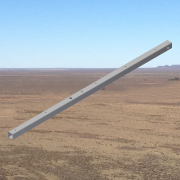
# Autodesk Inventor part: 2f2al
Saved by Autodesk Inventor 2014 SP1 (Build 180222100, 222)
## iProperties
Company: HERA Project
Created: 2013-06-27
Part Number: 2f2al
Material: Steel
Description: Feed backplane support crosspiece
Document SubType Name: Modeling
Designer: David DeBoer
Mass: 345.097 g
Surface Area: 540.887 cm^2
Volume: 43.9614 cm^3
Density: 7.85 g/cm^3
Appearance: Steel
Title: Feed backplane cross
Author: David DeBoer
Autodesk Inventor part; units mm, degrees
ref_plane "YZ Plane" through (0, 0, 0) normal (1, 0, 0) x (0, 1, 0)
ref_plane "XZ Plane" through (0, 0, 0) normal (0, 1, 0) x (-1, 0, 0)
ref_plane "XY Plane" through (0, 0, 0) normal (0, 0, 1) x (1, 0, 0)
sketch "Sketch1" plane through (0, 0, 0) normal (0, 0, 1) x (1, 0, 0)
  line L0 (3.175, 0) -> (22.225, 0)
  line L1 (25.4, 3.175) -> (25.4, 22.225)
  line L2 (22.225, 25.4) -> (3.175, 25.4)
  line L3 (0, 22.225) -> (0, 3.175)
  arc A0 (3.175, 25.4) -> (0, 22.225) centre (3.175, 22.225) ccw
  arc A1 (0, 3.175) -> (3.175, 0) centre (3.175, 3.175) ccw
  arc A2 (22.225, 0) -> (25.4, 3.175) centre (22.225, 3.175) ccw
  arc A3 (25.4, 22.225) -> (22.225, 25.4) centre (22.225, 22.225) ccw
  line L4 (3.175, 23.4) -> (22.225, 23.4)
  arc A4 (23.4, 22.225) -> (22.225, 23.4) centre (22.225, 22.225) ccw
  line L5 (23.4, 22.225) -> (23.4, 3.175)
  arc A5 (22.225, 2) -> (23.4, 3.175) centre (22.225, 3.175) ccw
  line L6 (22.225, 2) -> (3.175, 2)
  arc A6 (2, 3.175) -> (3.175, 2) centre (3.175, 3.175) ccw
  line L7 (2, 3.175) -> (2, 22.225)
  arc A7 (3.175, 23.4) -> (2, 22.225) centre (3.175, 22.225) ccw
  point P0 (0, 0)
  point P1 (25.4, 0)
  point P2 (0, 25.4)
  dimension "d0" = 25.4
  dimension "d1" = 25.4
  dimension "d2" = 3.175
  dimension "d3" = 2
  constraints: 16 end point, 16 point on circle, 8 centre point, 8 tangent, 6 point on line, 4 parallel, 3 equal radius, 2 perpendicular, 1 horizontal, 7 other
  measures "d0" distance of point (0, 0) point (25.4, 0)
  measures "d1" distance of point (0, 25.4) point (0, 0)
  measures "d2" radius of A0
  measures "d3" distance between parallel lines of L4 L2
extrude "Extrusion1" add sketch "Sketch1" along normal blind 1000
sketch "Sketch11" plane through (3.175, 25.4, 1000) normal (0, 1, 0) x (1, 0, 0)
  circle A0 centre (9.525, 500) radius 4.7917
  point P0 (-3.175, 1000)
  constraints: 1 centre point
hole "centerHole" at (12.7, 25.4, 500) direction (0, -1, 0) diameter 11 end through all clearance for "Flat Head Machine Screw" size "M10" standard "Ansi Metric M Profile"
sketch "Sketch12" plane through (3.175, 25.4, 1000) normal (0, 1, 0) x (1, 0, 0)
  line L0 (0, 1000) -> (0, 0) projected
  circle A0 centre (9.525, 927) radius 1.5875
  circle A1 centre (9.525, 777) radius 1.5875
  circle A2 centre (9.525, 627) radius 1.5875
  circle A3 centre (9.525, 500) radius 5.5 projected
  point P0 (-3.175, 1000)
  dimension "d76" = 3.175
  dimension "d80" = 150
  dimension "d140" = 127
  constraints: 3 centre point, 1 vertical, 4 other
  measures "d76" diameter of A0
  measures "d80" distance of A0.centre A1.centre
  measures "d140" distance of A2.centre A3.centre
hole "longSideHoles" at (12.7, 25.4, 73) at (12.7, 25.4, 223) at (12.7, 25.4, 373) direction (0, -1, 0) diameter 4.5 end through all clearance for "Flat Head Machine Screw" size "M4" standard "Ansi Metric M Profile"
sketch "Sketch13" plane through (3.175, 25.4, 1000) normal (0, 1, 0) x (1, 0, 0)
  line L0 (0, 1000) -> (0, 0) projected
  circle A0 centre (9.525, 68.2) radius 1.5875
  circle A1 centre (9.525, 220.6) radius 1.5875
  circle A2 centre (9.525, 373) radius 1.5875
  circle A3 centre (9.525, 500) radius 5.5 projected
  point P0 (-3.175, 1000)
  dimension "d96" = 152.4
  dimension "d137" = 127
  dimension "d138" = 152.4
  constraints: 3 centre point, 1 vertical, 4 other
  measures "d96" distance of A0.centre A1.centre
  measures "d137" distance of A2.centre A3.centre
  measures "d138" distance of A1.centre A2.centre
hole "shortSideHoles" at (12.7, 25.4, 627) at (12.7, 25.4, 779.4) at (12.7, 25.4, 931.8) direction (0, -1, 0) diameter 4.5 end through all clearance for "Flat Head Machine Screw" size "M4" standard "Ansi Metric M Profile"
sketch "Sketch14" plane through (25.4, 22.225, 1000) normal (1, 0, 0) x (0, 0, -1)
  line L0 (1000, -19.05) -> (1000, 0) projected
  line L1 (0, -19.05) -> (0, 0) projected
  circle A0 centre (30, -9.525) radius 4.7625
  circle A1 centre (980, -9.525) radius 4.7625
  point P0 (1000, -22.225)
  dimension "d108" = 9.525
  dimension "d109" = 30
  dimension "d110" = 9.525
  dimension "d111" = 20
  constraints: 2 centre point
  measures "d108" diameter of A0
  measures "d109" distance from line of L1 A0.centre
  measures "d110" diameter of A1
  measures "d111" distance from line of A1.centre L0
hole "shackleHole" at (25.4, 12.7, 970) at (25.4, 12.7, 20) direction (-1, 0, 0) diameter 8 end through all
sketch "Sketch15" plane through (3.175, 25.4, 1000) normal (0, 1, 0) x (1, 0, 0)
  circle A0 centre (9.525, 500) radius 5.5 projected
  circle A1 centre (9.525, 557.15) radius 3.175
  point P0 (-3.175, 1000)
  dimension "d119" = 6.35
  dimension "d120" = 57.15
  constraints: 1 centre point
  measures "d119" diameter of A1
  measures "d120" distance of A1.centre A0.centre
hole "collarHole" at (12.7, 25.4, 442.85) direction (0, -1, 0) diameter 6.6 end through all clearance for "Flat Head Machine Screw" size "M6" standard "Ansi Metric M Profile"
sketch "Sketch16" plane through (0, 0, 1000) normal (0, 0, 1) x (1, 0, 0)
  arc A0 (23.4, 22.225) -> (22.225, 23.4) centre (22.225, 22.225) ccw projected
  line L0 (23.4, 22.225) -> (23.4, 3.175) projected
  arc A1 (22.225, 2) -> (23.4, 3.175) centre (22.225, 3.175) ccw projected
  line L1 (22.225, 2) -> (3.175, 2) projected
  arc A2 (2, 3.175) -> (3.175, 2) centre (3.175, 3.175) ccw projected
  line L2 (2, 3.175) -> (2, 22.225) projected
  arc A3 (3.175, 23.4) -> (2, 22.225) centre (3.175, 22.225) ccw projected
  line L3 (3.175, 23.4) -> (22.225, 23.4) projected
  line L4 (0, 22.225) -> (0, 3.175) projected
  arc A4 (0, 3.175) -> (3.175, 0) centre (3.175, 3.175) ccw projected
  line L5 (3.175, 0) -> (22.225, 0) projected
  arc A5 (22.225, 0) -> (25.4, 3.175) centre (22.225, 3.175) ccw projected
  line L6 (25.4, 3.175) -> (25.4, 22.225) projected
  arc A6 (25.4, 22.225) -> (22.225, 25.4) centre (22.225, 22.225) ccw projected
  line L7 (22.225, 25.4) -> (3.175, 25.4) projected
  arc A7 (3.175, 25.4) -> (0, 22.225) centre (3.175, 22.225) ccw projected
  point P0 (0, 0)
extrude "removeSide" cut sketch "Sketch16" against normal blind 195
equation "\"d0\" = tube"
equation "\"d1\" = tube"
equation "\"tube\" = 25.4"
body "Solid1"
